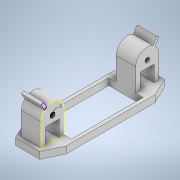
# Autodesk Inventor part: PalmWithBackstop
Saved by Autodesk Inventor 2021 (Build 250183000, 183)
## iProperties
Created: 2022-09-22
Part Number: PalmWithBackstop
Material: Generic
Document SubType Name: Modeling
Designer: ereg140
Density: 1 g/cm^3
Appearance: Default
Author: ereg140
Autodesk Inventor part; units mm, degrees
ref_plane "YZ Plane" through (0, 0, 0) normal (1, 0, 0) x (0, 1, 0)
ref_plane "XZ Plane" through (0, 0, 0) normal (0, 1, 0) x (-1, 0, 0)
ref_plane "XY Plane" through (0, 0, 0) normal (0, 0, 1) x (1, 0, 0)
sketch "Sketch1" plane through (0, 0, 0) normal (0, 1, 0) x (-1, 0, 0)
  line L0 (5.25, 27.1768) -> (-5.25, 27.1768)
  line L1 (-5.25, 27.1768) -> (-9, 19.3232)
  line L2 (-9, 19.3232) -> (-9, -19.3232)
  line L3 (-9, -19.3232) -> (-5.25, -27.1768)
  line L4 (-5.25, -27.1768) -> (5.25, -27.1768)
  line L5 (5.25, -27.1768) -> (9, -19.3232)
  line L6 (9, -19.3232) -> (9, 19.3232)
  line L7 (9, 19.3232) -> (5.25, 27.1768)
  line L8 (4.25, 25.6768) -> (-4.25, 25.6768)
  line L9 (-4.25, 25.6768) -> (-4.25, 19.3232)
  line L10 (-4.25, 19.3232) -> (4.25, 19.3232)
  line L11 (4.25, 19.3232) -> (4.25, 25.6768)
  line L12 (4.25, -19.3232) -> (-4.25, -19.3232)
  line L13 (-4.25, -19.3232) -> (-4.25, -25.6768)
  line L14 (-4.25, -25.6768) -> (4.25, -25.6768)
  line L15 (4.25, -25.6768) -> (4.25, -19.3232)
  point P0 (0, 0)
  point P1 (0, 22.5)
  point P2 (0, -22.5)
  point P3 (0, 25.6768)
  point P4 (0, 27.1768)
  point P5 (0, -25.6768)
  point P6 (0, -27.1768)
  point P7 (4.25, 22.5)
  point P8 (0, 19.3232)
  point P9 (0, -19.3232)
  point P10 (4.25, -22.5)
  point P11 (9, 0)
  dimension "d0" = 18
  dimension "d1" = 1.5
  dimension "d2" = 1.5
  dimension "d3" = 8.5
  dimension "d4" = 8.5
  dimension "d6" = 10.5
  dimension "d7" = 10.5
  dimension "d8" = 9
  dimension "d12" = 115.524
  dimension "d13" = 115.524
  dimension "d14" = 115.524
  dimension "d15" = 115.524
  dimension "d16" = 45
  constraints: 32 end point, 9 midpoint, 6 parallel, 6 vertical alignment, 5 horizontal alignment, 3 horizontal, 3 perpendicular
  measures "d0" distance between parallel lines of L2 L6
  measures "d1" distance between parallel lines of L8 L0
  measures "d2" distance between parallel lines of L4 L14
  measures "d3" distance of L13.end L14.end
  measures "d4" distance between parallel lines of L9 L11
  measures "d6" distance of L0.start L0.end
  measures "d7" distance of L3.end L4.end
  measures "d8" distance from line of point (0, 0) L6
  measures "d12" angle of L1 L0
  measures "d13" angle of L3 L4
  measures "d14" angle of L7 L0
  measures "d15" angle of L4 L5
  measures "d16" distance of point (0, -22.5) point (0, 22.5)
extrude "Extrusion1" add sketch "Sketch1" along normal blind 3 contours L7 L6 L5 L4 L3 L2 L1 L0 | L11 L10 L9 L8 | L15 L14 L13 L12
sketch "Sketch2" plane through (0, 3, 0) normal (0, 1, 0) x (1, 0, 0)
  line L0 (5.25, -27.1768) -> (9, -19.3232) projected
  line L1 (9, -19.3232) -> (9, 19.3232) projected
  line L2 (9, 19.3232) -> (5.25, 27.1768) projected
  line L3 (5.25, 27.1768) -> (-5.25, 27.1768) projected
  line L4 (-5.25, 27.1768) -> (-9, 19.3232) projected
  line L5 (-9, 19.3232) -> (-9, -19.3232) projected
  line L6 (-9, -19.3232) -> (-5.25, -27.1768) projected
  line L7 (-5.25, -27.1768) -> (5.25, -27.1768) projected
  line L8 (-4.25, -25.6768) -> (4.25, -25.6768)
  line L9 (4.25, -25.6768) -> (4.25, -15.6768)
  line L10 (4.25, -15.6768) -> (-4.25, -15.6768)
  line L11 (-4.25, -15.6768) -> (-4.25, -25.6768)
  line L12 (-4.25, 15.6768) -> (4.25, 15.6768)
  line L13 (4.25, 15.6768) -> (4.25, 25.6768)
  line L14 (4.25, 25.6768) -> (-4.25, 25.6768)
  line L15 (-4.25, 25.6768) -> (-4.25, 15.6768)
  point P0 (0, 0)
  point P1 (0, -25.6768)
  point P2 (0, -27.1768)
  dimension "d19" = 1.5
  dimension "d20" = 1.5
  dimension "d21" = 8.5
  dimension "d22" = 8.5
  dimension "d23" = 10
  dimension "d24" = 10
  constraints: 16 end point, 4 parallel, 2 horizontal, 2 midpoint, 2 perpendicular, 2 point on line, 1 vertical alignment
  measures "d19" distance between parallel lines of L8 L7
  measures "d20" distance between parallel lines of L3 L14
  measures "d21" distance of L8.start L8.end
  measures "d22" distance of L13.end L14.end
  measures "d23" distance of L10.end L8.start
  measures "d24" distance of L14.end L12.start
extrude "Extrusion2" add sketch "Sketch2" along normal blind 15 contours L11 L10 L9 L8 | L15 L14 L13 L12
fillet "Fillet1" radius 5 4 edges at (0, 18, 25.6768) (0, 18, 15.6768) (0, 18, -15.6768) (0, 18, -25.6768)
sketch "Sketch3" plane through (4.25, 3, 25.6768) normal (1, 0, 0) x (0, 0, -1)
  arc A0 (10, 10) -> (0, 10) centre (5, 10) ccw projected
  line L0 (0, 0) -> (0, 10) projected
  line L1 (10, 0) -> (0, 0) projected
  line L2 (10, 0) -> (10, 10) projected
  circle A1 centre (5, 10) radius 1
  arc A2 (10, 10) -> (0, 10) centre (5, 10) ccw projected
  line L3 (2.4906, 14.3247) -> (1.0669, 16.8692)
  line L4 (1.0669, 16.8692) -> (0, 16.2723)
  line L5 (0, 16.2723) -> (1.5075, 13.5781)
  arc A3 (2.4906, 14.3247) -> (1.5075, 13.5781) centre (5, 10) ccw
  point P0 (25.6768, -3)
  point P1 (1.5075, 13.5781)
  point P2 (2.4906, 14.3247)
  dimension "d28" = 2
  constraints: 6 end point, 4 point on circle, 2 centre point, 2 perpendicular, 1 coincident, 1 concentric
  measures "d28" diameter of A1
extrude "Extrusion3" add sketch "Sketch3" against normal up to surface (8.5 mm away) contours A0 L5 L4 L3
extrude "Extrusion4" cut sketch "Sketch3" against normal up to surface (8.5 mm away) contours A1
sketch "Sketch4" plane through (0, 3, 0) normal (0, 1, 0) x (1, 0, 0)
  line L0 (4.25, 15.6768) -> (-4.25, 15.6768) projected
  line L1 (-4.25, 15.6768) -> (-4.25, 25.6768) projected
  line L2 (-4.25, 25.6768) -> (4.25, 25.6768) projected
  line L3 (4.25, 25.6768) -> (4.25, 15.6768) projected
  line L4 (4.25, -25.6768) -> (-4.25, -25.6768) projected
  line L5 (-4.25, -25.6768) -> (-4.25, -15.6768) projected
  line L6 (-4.25, -15.6768) -> (4.25, -15.6768) projected
  line L7 (4.25, -15.6768) -> (4.25, -25.6768) projected
  line L8 (5.25, -27.1768) -> (9, -19.3232) projected
  line L9 (9, -19.3232) -> (9, 19.3232) projected
  line L10 (9, 19.3232) -> (5.25, 27.1768) projected
  line L11 (5.25, 27.1768) -> (-5.25, 27.1768) projected
  line L12 (-5.25, 27.1768) -> (-9, 19.3232) projected
  line L13 (-9, 19.3232) -> (-9, -19.3232) projected
  line L14 (-9, -19.3232) -> (-5.25, -27.1768) projected
  line L15 (-5.25, -27.1768) -> (5.25, -27.1768) projected
  line L16 (-7.5, 15.6768) -> (7.5, 15.6768)
  line L17 (7.5, 15.6768) -> (7.5, -15.6768)
  line L18 (7.5, -15.6768) -> (-7.5, -15.6768)
  line L19 (-7.5, -15.6768) -> (-7.5, 15.6768)
  point P0 (0, 0)
  dimension "d33" = 1.5
  dimension "d34" = 1.5
  constraints: 8 end point, 2 parallel, 1 horizontal, 1 perpendicular
  measures "d33" distance between parallel lines of L19 L13
  measures "d34" distance between parallel lines of L9 L17
extrude "Extrusion5" cut sketch "Sketch4" against normal up to surface (3 mm away) contours L16 L17 L18 L6 L19 L0
sketch "Sketch5" plane through (4.25, 3, 25.6768) normal (1, 0, 0) x (0, 0, -1)
  line L0 (6.3537, 0) -> (45, 0) projected
  line L1 (2, 7) -> (8, 7)
  line L2 (8, 7) -> (8, 0)
  line L3 (8, 0) -> (2, 0)
  line L4 (2, 0) -> (2, 7)
  line L5 (0, 0) -> (0, 10) projected
  line L6 (10, 0) -> (10, 10) projected
  circle A0 centre (5, 10) radius 1 projected
  point P0 (25.6768, -3)
  point P1 (6.3537, 0)
  dimension "d37" = 2
  dimension "d38" = 2
  dimension "d39" = 2
  constraints: 8 end point, 2 parallel, 1 horizontal, 1 perpendicular, 1 point on line
  measures "d37" distance between parallel lines of L4 L5
  measures "d38" distance between parallel lines of L6 L2
  measures "d39" distance edge to line of A0 L1
extrude "Extrusion6" cut sketch "Sketch5" against normal up to surface (8.5 mm away) contours L3 L4 L1 L2 L0
mirror "Mirror1" about plane through (0, 0, 0) normal (0, 0, 1) of "Extrusion3", "Extrusion6", "Extrusion4"
equation "\"d7\" = d6"
equation "\"d13\" = d12"
equation "\"d14\" = d12"
equation "\"d15\" = d12"
equation "\"d20\" = d19"
equation "\"d24\" = d23"
body "Solid1"
